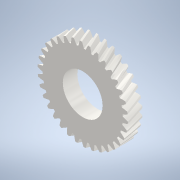
# Autodesk Inventor part: Цилиндрическое зубчатое зацепление1
Saved by Autodesk Inventor 2021 (Build 250183000, 183)
## iProperties
Created: 2021-03-22
Part Number: Цилиндрическое зубчатое зацепление1
Material: Steel
Document SubType Name: Modeling
Designer: Данил
Categories: <?xml version="1.0" encoding="UTF-16"?> <MemberInstance><Categories><FamilyTemplate><FamilyTemplateParameter ValueType="xs:double" Id="1" ObjectReferenceKey="da_z" ObjectType="kUserParameterObject"/><FamilyTemplateParameter ValueType="xs:double" Id="2" ObjectReferenceKey="da_b" ObjectType="kUserParameterObject"/><FamilyTemplateParameter ValueType="xs:double" Id="3" ObjectReferenceKey="da_beta" ObjectType="kUserParameterObject"/><FamilyTemplateParameter ValueType="xs:double" Id="4" ObjectReferenceKey="da_da" ObjectType="kUserParameterObject"/><FamilyTemplateParameter ValueType="xs:double" Id="5" ObjectReferenceKey="da_aw" ObjectType="kUserParameterObject"/><FamilyTemplateParameter ValueType="xs:string" Id="6" ObjectReferenceKey="EAIAABAAAACIAQAAAAAAAIAAAAAAAAAA" ObjectType="83910656" SubObjectId="SurfaceGeometry"/></FamilyTemplate><ParamToTemplateMap><ParamToTemplate CategoryParameter="//CategoryParameter[@InternalName='046C89C9-8512-4d59-83FE-43B91F4F132A']" TemplateParameter="1"/><ParamToTemplate CategoryParameter="//CategoryParameter[@InternalName='2552DF32-E462-4b46-AEBF-C6C7768E72AC']" TemplateParameter="2"/><ParamToTemplate CategoryParameter="//CategoryParameter[@InternalName='C9EE641D-15FC-4fae-A226-E94C4372FDD7']" TemplateParameter="3"/><ParamToTemplate><ParamToTemplate CategoryParameter="//CategoryParameter[@InternalName='00B6519A-459B-49c7-AD84-2E56D39A5744']" ConstantValue="0.000000"/></ParamToTemplate><ParamToTemplate><ParamToTemplate CategoryParameter="//CategoryParameter[@InternalName='04B31F0E-C7A6-4894-AA32-9629BEFACF47']" ConstantValue="1.000000"/></ParamToTemplate><ParamToTemplate><ParamToTemplate CategoryParameter="//CategoryParameter[@InternalName='43CBEC2E-7847-49e7-A936-2F7889FCB2D9']" ConstantValue="0.250000"/></ParamToTemplate><ParamToTemplate><ParamToTemplate CategoryParameter="//CategoryParameter[@InternalName='B1EFC894-105D-4ebd-86BF-FA20ED196853']" ConstantValue="0.300000"/></ParamToTemplate><ParamToTemplate><ParamToTemplate CategoryParameter="//CategoryParameter[@InternalName='51175063-3D10-4879-93E8-6246FE8B403D']" ConstantValue="2060000000.000000"/></ParamToTemplate><ParamToTemplate><ParamToTemplate CategoryParameter="//CategoryParameter[@InternalName='A3A52E27-4454-46a9-B0BD-C932399B70AF']" ConstantValue="0.300000"/></ParamToTemplate><ParamToTemplate><ParamToTemplate CategoryParameter="//CategoryParameter[@InternalName='91B76062-C214-41d9-B1B9-14D2AB99603D']" ConstantValue="0.350000"/></ParamToTemplate><ParamToTemplate><ParamToTemplate CategoryParameter="//CategoryParameter[@InternalName='374E806E-8B8A-4dda-A9AA-1039D6500AD2']" ConstantValue="2.857143"/></ParamToTemplate><ParamToTemplate><ParamToTemplate CategoryParameter="//CategoryParameter[@InternalName='2D373A89-B862-43d6-8D0B-0CBF12AB9F6C']" ConstantValue="0.349066"/></ParamToTemplate><ParamToTemplate CategoryParameter="//CategoryParameter[@InternalName='37777632-D6A2-4fac-9D53-DB8ACD95C989']" TemplateParameter="4"/><ParamToTemplate CategoryParameter="//CategoryParameter[@InternalName='FD1017F1-B727-4f7e-9707-0F86F1FF9423']" TemplateParameter="5"/><ParamToTemplate><ParamToTemplate CategoryParameter="//CategoryParameter[@InternalName='9E1B4470-B2D3-4ff1-B813-535BB4CDF51A']" ConstantValue="3520000.000000"/></ParamToTemplate><ParamToTemplate><ParamToTemplate CategoryParameter="//CategoryParameter[@InternalName='F8452263-BFF6-458c-9FB1-07C4B99E95CD']" ConstantValue="11400000.000000"/></ParamToTemplate><ParamToTemplate><ParamToTemplate CategoryParameter="//CategoryParameter[@InternalName='3E3BB259-FD49-497f-8171-6EBC954A3479']" ConstantValue="2.000000"/></ParamToTemplate><ParamToTemplate CategoryParameter="//CategoryParameter[@InternalName='27C3BAF2-7550-4e4b-AE2C-0DB134B7D9B7']" TemplateParameter="6"/></ParamToTemplateMap><Category DisplayName="Gear" InternalName="DC85795E-93AB-48d5-8EEE-5A27447B64BD" Mnemonic="Gear"><CategoryParameter DisplayName="z" InternalName="046C89C9-8512-4d59-83FE-43B91F4F132A" Mnemonic="z"/><CategoryParameter DisplayName="b" InternalName="2552DF32-E462-4b46-AEBF-C6C7768E72AC" Mnemonic="b"/><CategoryParameter DisplayName="||b|" InternalName="C9EE641D-15FC-4fae-A226-E94C4372FDD7" Mnemonic="beta"/><CategoryParameter DisplayName="x" InternalName="00B6519A-459B-49c7-AD84-2E56D39A5744" Mnemonic="x"/><CategoryParameter DisplayName="a*" InternalName="04B31F0E-C7A6-4894-AA32-9629BEFACF47" Mnemonic="a"/><CategoryParameter DisplayName="c*" InternalName="43CBEC2E-7847-49e7-A936-2F7889FCB2D9" Mnemonic="c"/><CategoryParameter DisplayName="r|.f|*" InternalName="B1EFC894-105D-4ebd-86BF-FA20ED196853" Mnemonic="rf"/><CategoryParameter DisplayName="E" InternalName="51175063-3D10-4879-93E8-6246FE8B403D" Mnemonic="E"/><CategoryParameter DisplayName="||m|" InternalName="A3A52E27-4454-46a9-B0BD-C932399B70AF" Mnemonic="mi"/><Category DisplayName="SpurGear" InternalName="26C5A22E-A91E-4dfd-A3B3-23CCAFAE1764" Mnemonic="SpurGear"><CategoryParameter DisplayName="m" InternalName="91B76062-C214-41d9-B1B9-14D2AB99603D" Mnemonic="m"/><CategoryParameter DisplayName="P" InternalName="374E806E-8B8A-4dda-A9AA-1039D6500AD2" Mnemonic="PP"/><CategoryParameter DisplayName="||a|" InternalName="2D373A89-B862-43d6-8D0B-0CBF12AB9F6C" Mnemonic="alpha"/><CategoryParameter DisplayName="d|.a|" InternalName="37777632-D6A2-4fac-9D53-DB8ACD95C989" Mnemonic="da"/><CategoryParameter DisplayName="a|.w|" InternalName="FD1017F1-B727-4f7e-9707-0F86F1FF9423" Mnemonic="aw"/><CategoryParameter DisplayName="||s||.Flim|" InternalName="9E1B4470-B2D3-4ff1-B813-535BB4CDF51A" Mnemonic="sFlim"/><CategoryParameter DisplayName="||s||.Hlim|" InternalName="F8452263-BFF6-458c-9FB1-07C4B99E95CD" Mnemonic="sHlim"/><CategoryParameter DisplayName="тип" InternalName="3E3BB259-FD49-497f-8171-6EBC954A3479" Mnemonic="type"/><CategoryParameter DisplayName="PitchDiameter" InternalName="27C3BAF2-7550-4e4b-AE2C-0DB134B7D9B7" Mnemonic="IDS_PITCHDIAM"/></Category></Category></Categories></MemberInstance>
Density: 1 g/cm^3
Appearance: Steel
CustomPartVersion: 1
Author: Данил
Autodesk Inventor part; units mm, degrees
ref_plane "YZ Plane" through (0, 0, 0) normal (1, 0, 0) x (0, 1, 0)
ref_plane "XZ Plane" through (0, 0, 0) normal (0, 1, 0) x (-1, 0, 0)
ref_plane "XY Plane" through (0, 0, 0) normal (0, 0, 1) x (1, 0, 0)
sketch "Sketch1" plane through (0, 0, 0) normal (0, 0, 1) x (1, 0, 0)
  circle A0 centre (0, 0) radius 68.1384
  dimension "d0" = 136.2769
  constraints: 1 centre point
  measures "d0" diameter of A0
extrude "Extrusion1" add sketch "Sketch1" along normal blind 22
ref_plane "Work Plane2" through (0, 0, 11) normal (0, 0, 1) x (1, 0, 0)
sketch "Sketch2" plane through (0, 0, 0) normal (0, 0, -1) x (-1, 0, 0)
  circle A0 centre (0, 0) radius 68.1384 projected
  circle A1 centre (0, 0) radius 64.6384
  dimension "d3" = 129.2769
  constraints: 1 centre point, 1 coincident
  measures "d3" diameter of A1
surface extrude "Средний диаметр" sketch "Sketch2" against normal through all shown no curves A1
ref_plane "Work Plane8" through (0, 0, 0) normal (0.9957342, 0.0922684, 0) x (0, 0, 1)
ref_plane "Work Plane9" through (0, 0, 0) normal (1, 0, 0) x (0, 1, 0)
spur gear teeth "Цилиндрическое зубчатое зацепление" teeth 34 pitch diameter 129.2769 tip diameter 136.2769 root diameter 120.5269 face width 22 helix angle 23 hand left start plane through (0, 0, 0) normal (0, 0, -1) x (-1, 0, 0)
sketch "Эскиз3" plane through (0, 0, 22) normal (0, 0, 1) x (1, 0, 0)
  circle A0 centre (0, 0) radius 30
  dimension "d49" = 60
  constraints: 1 centre point, 1 coincident
  measures "d49" diameter of A0
extrude "Выдавливание2" cut sketch "Эскиз3" against normal through all
chamfer "Фаска1" distance 1 angle 45 34 edges at (22.0328, 64.4779, 22) (33.5055, 59.3315, 22) (43.8371, 52.1647, 22) (52.6759, 43.2214, 22) (59.7209, 32.8063, 22) (64.7322, 21.2741, 22) (67.5391, 9.0173, 22) (68.0461, -3.5465, 22) (66.2358, -15.9896, 22) (62.1699, -27.8881, 22) (55.9869, -38.837, 22) (47.8974, -48.4633, 22) (38.1767, -56.4392, 22) (27.156, -62.4932, 22) (15.2106, -66.419, 22) (2.7471, -68.083, 22) (-9.8099, -67.4286, 22) (-22.0328, -64.4779, 22) (-33.5055, -59.3315, 22) (-43.8371, -52.1647, 22) (-52.6759, -43.2214, 22) (-59.7209, -32.8063, 22) (-64.7322, -21.2741, 22) (-67.5391, -9.0173, 22) (-68.0461, 3.5465, 22) (-66.2358, 15.9896, 22) (-62.1699, 27.8881, 22) (-55.9869, 38.837, 22) (-47.8974, 48.4633, 22) (-38.1767, 56.4392, 22) (-27.156, 62.4932, 22) (-15.2106, 66.419, 22) (-2.7471, 68.083, 22) (9.8099, 67.4286, 22) measured on face at (-33.2596, -58.8962, 22) measured on face at (-67.0435, -8.9511, 22) measured on face at (-67.5468, 3.5205, 22) measured on face at (-21.8711, -64.0048, 22) measured on face at (64.2572, 21.1179, 22) measured on face at (26.9568, -62.0346, 22) measured on face at (-37.8966, 56.0251, 22) measured on face at (-9.7379, -66.9338, 22) measured on face at (-64.2572, -21.1179, 22) measured on face at (-61.7137, 27.6835, 22) measured on face at (47.5459, -48.1076, 22) measured on face at (-15.0989, 65.9316, 22) measured on face at (-59.2827, -32.5656, 22) measured on face at (-47.5459, 48.1076, 22) measured on face at (9.7379, 66.9338, 22) measured on face at (-43.5154, -51.7819, 22) measured on face at (15.0989, -65.9316, 22) measured on face at (43.5154, 51.7819, 22) measured on face at (67.0435, 8.9511, 22) measured on face at (33.2596, 58.8962, 22) measured on face at (2.727, -67.5834, 22) measured on face at (-52.2894, -42.9043, 22) measured on face at (-55.5761, 38.552, 22) measured on face at (-2.727, 67.5834, 22) measured on face at (59.2827, 32.5656, 22) measured on face at (37.8966, -56.0251, 22) measured on face at (-65.7498, 15.8722, 22) measured on face at (61.7137, -27.6835, 22) measured on face at (65.7498, -15.8722, 22) measured on face at (55.5761, -38.552, 22) measured on face at (21.8711, 64.0048, 22) measured on face at (67.5468, -3.5205, 22) measured on face at (52.2894, 42.9043, 22) measured on face at (-26.9568, 62.0346, 22)
chamfer "Фаска2" distance 1 angle 45 34 edges at (12.5204, 66.9783, 0) (0, 68.1384, 0) (-12.5204, 66.9783, 0) (-24.6144, 63.5372, 0) (-35.8703, 57.9325, 0) (-45.9046, 50.3549, 0) (-54.3757, 41.0626, 0) (-60.995, 30.3719, 0) (-65.5373, 18.647, 0) (-67.8478, 6.287, 0) (-67.8478, -6.287, 0) (-65.5373, -18.647, 0) (-60.995, -30.3719, 0) (-54.3757, -41.0626, 0) (-45.9046, -50.3549, 0) (-35.8703, -57.9325, 0) (-24.6144, -63.5372, 0) (-12.5204, -66.9783, 0) (0, -68.1384, 0) (12.5204, -66.9783, 0) (24.6144, -63.5372, 0) (35.8703, -57.9325, 0) (45.9046, -50.3549, 0) (54.3757, -41.0626, 0) (60.995, -30.3719, 0) (65.5373, -18.647, 0) (67.8478, -6.287, 0) (67.8478, 6.287, 0) (65.5373, 18.647, 0) (60.995, 30.3719, 0) (54.3757, 41.0626, 0) (45.9046, 50.3549, 0) (35.8703, 57.9325, 0) (24.6144, 63.5372, 0) measured on face at (-65.0564, 18.5101, 0) measured on face at (-35.6071, -57.5074, 0) measured on face at (12.4285, -66.4868, 0) measured on face at (-67.3499, 6.2409, 0) measured on face at (-60.5475, -30.149, 0) measured on face at (45.5677, -49.9854, 0) measured on face at (60.5475, -30.149, 0) measured on face at (24.4338, 63.071, 0) measured on face at (-45.5677, -49.9854, 0) measured on face at (53.9766, 40.7613, 0) measured on face at (12.4285, 66.4868, 0) measured on face at (60.5475, 30.149, 0) measured on face at (0, -67.6384, 0) measured on face at (-53.9766, -40.7613, 0) measured on face at (-60.5475, 30.149, 0) measured on face at (-24.4338, -63.071, 0) measured on face at (35.6071, 57.5074, 0) measured on face at (67.3499, -6.2409, 0) measured on face at (35.6071, -57.5074, 0) measured on face at (67.3499, 6.2409, 0) measured on face at (65.0564, 18.5101, 0) measured on face at (-65.0564, -18.5101, 0) measured on face at (-45.5677, 49.9854, 0) measured on face at (53.9766, -40.7613, 0) measured on face at (0, 67.6384, 0) measured on face at (-24.4338, 63.071, 0) measured on face at (-12.4285, -66.4868, 0) measured on face at (24.4338, -63.071, 0) measured on face at (45.5677, 49.9854, 0) measured on face at (-53.9766, 40.7613, 0) measured on face at (-35.6071, 57.5074, 0) measured on face at (-67.3499, -6.2409, 0) measured on face at (65.0564, -18.5101, 0) measured on face at (-12.4285, 66.4868, 0)
equation "\"d0\" = da_da"
equation "\"d1\" = da_b"
equation "\"d3\" = da_d"
equation "\"d16\" = da_aw"
equation "\"d43\" = da_aw"
equation "\"d46\" = da_aw"
equation "\"da_da\" = 136.276885"
equation "\"da_b\" = 22"
equation "\"da_d\" = 129.276885"
equation "\"da_aw\" = 201.51985"
body "Solid1"
body "Srf1"
